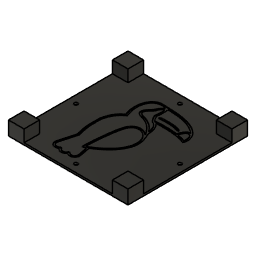
base (Autodesk Fusion 360 design; units mm, degrees)
Autodesk Fusion 360 part; units mm, degrees
sketch "Sketch1" plane through (0, 0, 0) normal (0, 0, 1) x (1, 0, 0)
  line L0 (-50, 50) -> (50, 50)
  line L1 (50, 50) -> (50, -50)
  line L2 (50, -50) -> (-50, -50)
  line L3 (-50, -50) -> (-50, 50)
  dimension "d73" = 100
  constraint horizontal L0
  constraint vertical L1
  constraint horizontal L2
  constraint vertical L3
  measures "d73" distance of L0.start L0.end
extrude "Extrude1" add sketch "Sketch1" along normal blind 1.6
sketch "Sketch2" plane through (0, 0, 1.6) normal (0, 0, 1) x (-1, 0, 0)
  line L0 (50, 50) -> (-50, 50)
  line L1 (-50, 50) -> (-50, -50)
  line L2 (-50, -50) -> (50, -50)
  line L3 (50, -50) -> (50, 50)
  line L4 (50, -50) -> (37, -50)
  line L5 (37, -50) -> (37, -37)
  line L6 (37, -37) -> (50, -37)
  line L7 (50, -37) -> (50, -50)
  dimension "d3" = 13
  dimension "d4" = 13
  constraint horizontal L4
  constraint vertical L5
  constraint horizontal L6
  constraint vertical L7
  constraint coincident L2.end L3.start
  measures "d3" distance of L2.end L4.end
  measures "d4" distance of L2.end L6.end
extrude "Extrude2" add sketch "Sketch2" along normal blind 10 contours L2 L3 L4 L5 L6 L7
sketch "Sketch3" plane through (0, 0, 1.6) normal (0, 0, 1) x (-1, 0, 0)
  line L0 (37, -50) -> (37, -37)
  line L1 (37, -37) -> (50, -37)
  line L2 (50, -37) -> (50, 50)
  line L3 (50, 50) -> (-50, 50)
  line L4 (-50, 50) -> (-50, -50)
  line L5 (-50, -50) -> (37, -50)
  line L6 (50, 50) -> (37, 50)
  line L7 (37, 50) -> (37, 37)
  line L8 (37, 37) -> (50, 37)
  line L9 (50, 37) -> (50, 50)
  dimension "d7" = 13
  dimension "d8" = 13
  constraint horizontal L6
  constraint vertical L7
  constraint horizontal L8
  constraint vertical L9
  constraint coincident L2.end L3.start
  measures "d7" distance of L2.end L6.end
  measures "d8" distance of L2.end L8.end
extrude "Extrude3" add sketch "Sketch3" along normal blind 10 contours L2 L3 L6 L7 L8 L9
sketch "Sketch4" plane through (0, 0, 1.6) normal (0, 0, 1) x (-1, 0, 0)
  line L0 (37, 37) -> (37, 50)
  line L1 (37, 50) -> (-50, 50)
  line L2 (-50, 50) -> (-50, -50)
  line L3 (-50, -50) -> (37, -50)
  line L4 (37, -50) -> (37, -37)
  line L5 (37, -37) -> (50, -37)
  line L6 (50, -37) -> (50, 37)
  line L7 (50, 37) -> (37, 37)
  line L8 (-50, 50) -> (-37, 50)
  line L9 (-37, 50) -> (-37, 37)
  line L10 (-37, 37) -> (-50, 37)
  line L11 (-50, 37) -> (-50, 50)
  dimension "d11" = 13
  dimension "d12" = 13
  constraint horizontal L8
  constraint vertical L9
  constraint horizontal L10
  constraint vertical L11
  constraint coincident L1.end L2.start
  measures "d11" distance of L1.end L8.end
  measures "d12" distance of L1.end L10.end
extrude "Extrude4" add sketch "Sketch4" along normal blind 10 contours L1 L2 L8 L9 L10 L11
sketch "Sketch5" plane through (0, 0, 1.6) normal (0, 0, 1) x (-1, 0, 0)
  line L0 (-37, 50) -> (-37, 37)
  line L1 (-37, 37) -> (-50, 37)
  line L2 (-50, 37) -> (-50, -50)
  line L3 (-50, -50) -> (37, -50)
  line L4 (37, -50) -> (37, -37)
  line L5 (37, -37) -> (50, -37)
  line L6 (50, -37) -> (50, 37)
  line L7 (50, 37) -> (37, 37)
  line L8 (37, 37) -> (37, 50)
  line L9 (37, 50) -> (-37, 50)
  line L10 (-50, -50) -> (-37, -50)
  line L11 (-37, -50) -> (-37, -37)
  line L12 (-37, -37) -> (-50, -37)
  line L13 (-50, -37) -> (-50, -50)
  dimension "d15" = 13
  dimension "d16" = 13
  constraint horizontal L10
  constraint vertical L11
  constraint horizontal L12
  constraint vertical L13
  constraint coincident L2.end L3.start
  measures "d15" distance of L2.end L10.end
  measures "d16" distance of L2.end L12.end
extrude "Extrude5" add sketch "Sketch5" along normal blind 10 contours L2 L3 L10 L11 L12 L13
sketch "Sketch15" plane through (0, 0, 1.6) normal (0, 0, 1) x (1, 0, 0)
  line L0 (-40, 50) -> (-50, 50)
  line L1 (-50, -50) -> (-40, -50)
  line L2 (-50, -40) -> (-50, -50)
  line L3 (50, -50) -> (50, -40)
  line L4 (40, -50) -> (50, -50)
  line L5 (50, 50) -> (40, 50)
  line L6 (-50, 50) -> (-50, 40)
  line L7 (50, 40) -> (50, 50)
  line L8 (40, 50) -> (-40, 50)
  line L9 (50, -40) -> (50, 40)
  line L10 (-40, -50) -> (40, -50)
  line L11 (-50, 40) -> (-50, -40)
  line L12 (37, 37) -> (37, 50)
  line L13 (37, 50) -> (-37, 50)
  line L14 (-37, 50) -> (-37, 37)
  line L15 (-37, 37) -> (-50, 37)
  line L16 (-50, 37) -> (-50, -37)
  line L17 (-50, -37) -> (-37, -37)
  line L18 (-37, -37) -> (-37, -50)
  line L19 (-37, -50) -> (37, -50)
  line L20 (37, -50) -> (37, -37)
  line L21 (37, -37) -> (50, -37)
  line L22 (50, -37) -> (50, 37)
  line L23 (50, 37) -> (37, 37)
  point P0 (-43.5004, 0.0001)
  point P1 (0.0001, 43.5004)
  point P2 (43.5004, -0.0001)
  point P3 (-0.0001, -43.5004)
  dimension "d36" = 50
  dimension "d38" = 50
  dimension "d40" = 50
  dimension "d43" = 50
  dimension "d45" = 6.5
  dimension "d47" = 6.5
  dimension "d49" = 6.5
  dimension "d51" = 6.5
  measures "d36" distance of P0 L0
  measures "d38" distance of P3 L2
  measures "d40" distance of P2 L4
  measures "d43" distance of P1 L7
  measures "d45" distance of P1 L8
  measures "d47" distance of P2 L9
  measures "d49" distance of P3 L10
  measures "d51" distance of P0 L11
hole "Hole1" at (-0.0001, -43.5004, 1.6711) at (-43.5004, 0.0001, 1.6711) at (43.5004, -0.0001, 1.6711) at (0.0001, 43.5004, 1.6711) direction (0, 0, -1) diameter 3 depth 15 tip angle 118
sketch "Sketch16" plane through (0, 0, 0) normal (0, 0, 1) x (1, 0, 0)
  spline S0 degree 3 poles (-9.4935, 35.6608) (-16.0287, 33.5706) (-18.8069, 24.1515) (-15.6848, 14.891) knots 0 0 0 0 1 1 1 1
  spline S1 degree 3 poles (-15.6848, 14.891) (-15.3673, 13.965) (-15.1292, 13.1977) (-15.1821, 13.1713) knots 0 0 0 0 1 1 1 1
  spline S2 degree 3 poles (-15.1821, 13.1713) (-18.5158, 10.9752) (-21.241, 6.8477) (-22.5904, 2.0323) knots 0 0 0 0 1 1 1 1
  spline S3 degree 3 poles (-22.5904, 2.0323) (-23.1196, 0.1537) (-23.1725, -0.7194) (-23.1725, -5.6406) knots 0 0 0 0 1 1 1 1
  spline S4 degree 3 poles (-23.1725, -5.6406) (-23.1725, -11.4615) (-22.9608, -13.3929) (-21.6115, -18.9227) knots 0 0 0 0 1 1 1 1
  line L0 (-21.6115, -18.9227) -> (-21.0029, -21.4627)
  line L1 (-21.0029, -21.4627) -> (-23.1196, -28.6065)
  spline S5 degree 3 poles (-23.1196, -28.6065) (-24.6277, -33.7129) (-25.1833, -35.9883) (-25.0775, -36.5704) knots 0 0 0 0 1 1 1 1
  spline S6 degree 3 poles (-25.0775, -36.5704) (-24.8394, -37.761) (-23.9927, -39.031) (-23.0137, -39.6396) knots 0 0 0 0 1 1 1 1
  spline S7 degree 3 poles (-23.0137, -39.6396) (-21.9554, -40.2746) (-19.7329, -40.354) (-18.9127, -39.7719) knots 0 0 0 0 1 1 1 1
  spline S8 degree 3 poles (-18.9127, -39.7719) (-18.3835, -39.4015) (-18.2777, -39.4279) (-17.5633, -40.1423) knots 0 0 0 0 1 1 1 1
  spline S9 degree 3 poles (-17.5633, -40.1423) (-15.9758, -41.7563) (-13.33, -41.7298) (-11.7954, -40.1423) knots 0 0 0 0 1 1 1 1
  spline S10 degree 3 poles (-11.7954, -40.1423) (-11.1075, -39.4279) (-11.0281, -39.4015) (-10.5783, -39.8248) knots 0 0 0 0 1 1 1 1
  spline S11 degree 3 poles (-10.5783, -39.8248) (-9.9433, -40.3804) (-7.6679, -40.5921) (-6.6625, -40.1688) knots 0 0 0 0 1 1 1 1
  spline S12 degree 3 poles (-6.6625, -40.1688) (-5.5512, -39.719) (-4.3342, -38.2373) (-4.1225, -37.0996) knots 0 0 0 0 1 1 1 1
  spline S13 degree 3 poles (-4.1225, -37.0996) (-3.9902, -36.4117) (-4.2283, -34.7448) (-4.9162, -31.4904) knots 0 0 0 0 1 1 1 1
  spline S14 degree 3 poles (-4.9162, -31.4904) (-5.4454, -28.9504) (-5.8423, -26.8338) (-5.8158, -26.8338) knots 0 0 0 0 1 1 1 1
  spline S15 degree 3 poles (-5.8158, -26.8338) (-5.7629, -26.8073) (-4.5458, -26.0135) (-3.0906, -25.0346) knots 0 0 0 0 1 1 1 1
  spline S16 degree 3 poles (-3.0906, -25.0346) (4.5029, -19.981) (9.7681, -13.4458) (11.3821, -7.0429) knots 0 0 0 0 1 1 1 1
  spline S17 degree 3 poles (11.3821, -7.0429) (12.1229, -4.0796) (11.9642, -0.296) (11.0117, 2.1646) knots 0 0 0 0 1 1 1 1
  spline S18 degree 3 poles (11.0117, 2.1646) (10.6148, 3.1171) (10.1915, 4.3606) (10.0063, 4.9427) knots 0 0 0 0 1 1 1 1
  spline S19 degree 3 poles (10.0063, 4.9427) (9.821, 5.5248) (9.3977, 6.5302) (9.0538, 7.1652) knots 0 0 0 0 1 1 1 1
  spline S20 degree 3 poles (9.0538, 7.1652) (8.6569, 7.906) (8.4188, 8.7527) (8.4188, 9.5465) knots 0 0 0 0 1 1 1 1
  spline S21 degree 3 poles (8.4188, 9.5465) (8.3923, 12.8008) (7.0165, 16.5315) (5.2173, 18.1719) knots 0 0 0 0 1 1 1 1
  spline S22 degree 3 poles (5.2173, 18.1719) (4.6088, 18.701) (4.1854, 19.2037) (4.2648, 19.2831) knots 0 0 0 0 1 1 1 1
  spline S23 degree 3 poles (4.2648, 19.2831) (4.3442, 19.336) (7.0165, 19.389) (10.1915, 19.389) knots 0 0 0 0 1 1 1 1
  spline S24 degree 3 poles (10.1915, 19.389) (17.8644, 19.389) (24.5054, 18.4894) (27.8656, 17.0077) knots 0 0 0 0 1 1 1 1
  spline S25 degree 3 poles (27.8656, 17.0077) (28.4742, 16.7431) (29.1092, 16.5844) (29.2679, 16.6902) knots 0 0 0 0 1 1 1 1
  spline S26 degree 3 poles (29.2679, 16.6902) (29.7442, 16.9812) (30.194, 19.6006) (30.0088, 21.0029) knots 0 0 0 0 1 1 1 1
  spline S27 degree 3 poles (30.0088, 21.0029) (29.1356, 27.4588) (22.4946, 32.4329) (12.0965, 34.3908) knots 0 0 0 0 1 1 1 1
  spline S28 degree 3 poles (12.0965, 34.3908) (8.604, 35.0788) (7.281, 35.211) (1.1427, 35.555) knots 0 0 0 0 1 1 1 1
  spline S29 degree 3 poles (1.1427, 35.555) (-7.5621, 36.0312) (-8.3294, 36.0312) (-9.4935, 35.6608) knots 0 0 0 0 1 1 1 1
  spline S30 degree 3 poles (-4.3342, 34.5496) (-2.9054, 34.3644) (-2.5879, 33.9675) (-3.3817, 33.3325) knots 0 0 0 0 1 1 1 1
  spline S31 degree 3 poles (-3.3817, 33.3325) (-4.8898, 32.1419) (-5.5777, 31.2423) (-6.1069, 29.7871) knots 0 0 0 0 1 1 1 1
  spline S32 degree 3 poles (-6.1069, 29.7871) (-6.5567, 28.57) (-7.0858, 27.8027) (-8.3029, 26.6121) knots 0 0 0 0 1 1 1 1
  spline S33 degree 3 poles (-8.3029, 26.6121) (-10.1815, 24.76) (-10.9487, 23.4106) (-10.9752, 21.8231) knots 0 0 0 0 1 1 1 1
  spline S34 degree 3 poles (-10.9752, 21.8231) (-11.0017, 19.7329) (-9.6787, 18.6217) (-6.1862, 17.7485) knots 0 0 0 0 1 1 1 1
  spline S35 degree 3 poles (-6.1862, 17.7485) (-2.535, 16.8225) (1.1163, 14.7588) (3.5504, 12.1658) knots 0 0 0 0 1 1 1 1
  spline S36 degree 3 poles (3.5504, 12.1658) (4.9263, 10.7371) (7.6779, 7.1652) (7.5192, 7.0065) knots 0 0 0 0 1 1 1 1
  spline S37 degree 3 poles (7.5192, 7.0065) (7.4663, 6.9535) (6.9106, 7.271) (6.2756, 7.6944) knots 0 0 0 0 1 1 1 1
  spline S38 degree 3 poles (6.2756, 7.6944) (4.7675, 8.7262) (2.1481, 9.4142) (0.5077, 9.176) knots 0 0 0 0 1 1 1 1
  spline S39 degree 3 poles (0.5077, 9.176) (-2.244, 8.7792) (-4.4665, 7.0858) (-5.71, 4.44) knots 0 0 0 0 1 1 1 1
  spline S40 degree 3 poles (-5.71, 4.44) (-7.6679, 0.286) (-9.2025, -10.2179) (-9.9962, -24.8758) knots 0 0 0 0 1 1 1 1
  spline S41 degree 3 poles (-9.9962, -24.8758) (-10.155, -27.9715) (-10.1285, -28.2625) (-9.7052, -28.4477) knots 0 0 0 0 1 1 1 1
  spline S42 degree 3 poles (-9.7052, -28.4477) (-9.3877, -28.5535) (-8.8321, -28.3948) (-8.1971, -28.0244) knots 0 0 0 0 1 1 1 1
  spline S43 degree 3 poles (-8.1971, -28.0244) (-7.4562, -27.601) (-7.1652, -27.5481) (-7.0858, -27.7863) knots 0 0 0 0 1 1 1 1
  spline S44 degree 3 poles (-7.0858, -27.7863) (-7.0329, -27.9715) (-6.6096, -30.0088) (-6.1598, -32.2842) knots 0 0 0 0 1 1 1 1
  spline S45 degree 3 poles (-6.1598, -32.2842) (-5.3925, -36.1206) (-5.3396, -36.5175) (-5.71, -37.3642) knots 0 0 0 0 1 1 1 1
  spline S46 degree 3 poles (-5.71, -37.3642) (-6.4773, -39.1633) (-8.6733, -39.6396) (-10.1815, -38.3167) knots 0 0 0 0 1 1 1 1
  spline S47 degree 3 poles (-10.1815, -38.3167) (-11.3192, -37.3377) (-11.5837, -37.3377) (-12.0865, -38.2902) knots 0 0 0 0 1 1 1 1
  spline S48 degree 3 poles (-12.0865, -38.2902) (-12.6156, -39.3485) (-13.4887, -39.9042) (-14.5471, -39.9042) knots 0 0 0 0 1 1 1 1
  spline S49 degree 3 poles (-14.5471, -39.9042) (-15.6583, -39.9042) (-16.9019, -39.2692) (-17.1135, -38.6077) knots 0 0 0 0 1 1 1 1
  spline S50 degree 3 poles (-17.1135, -38.6077) (-17.431, -37.5758) (-17.9073, -37.47) (-18.9656, -38.1844) knots 0 0 0 0 1 1 1 1
  spline S51 degree 3 poles (-18.9656, -38.1844) (-21.0294, -39.5867) (-23.5694, -38.5019) (-23.5958, -36.2) knots 0 0 0 0 1 1 1 1
  spline S52 degree 3 poles (-23.5958, -36.2) (-23.5958, -35.6973) (-22.6962, -32.1783) (-21.585, -28.3948) knots 0 0 0 0 1 1 1 1
  line L2 (-21.585, -28.3948) -> (-19.5742, -21.5156)
  line L3 (-19.5742, -21.5156) -> (-20.2356, -18.6052)
  spline S53 degree 3 poles (-20.2356, -18.6052) (-21.585, -12.9167) (-21.8496, -10.6942) (-21.8496, -5.5083) knots 0 0 0 0 1 1 1 1
  spline S54 degree 3 poles (-21.8496, -5.5083) (-21.8231, -1.3544) (-21.7437, -0.296) (-21.2675, 1.5031) knots 0 0 0 0 1 1 1 1
  spline S55 degree 3 poles (-21.2675, 1.5031) (-20.315, 4.9692) (-18.8069, 7.7208) (-16.6373, 9.9433) knots 0 0 0 0 1 1 1 1
  spline S56 degree 3 poles (-16.6373, 9.9433) (-15.579, 11.0017) (-14.4412, 12.0335) (-14.0708, 12.2717) knots 0 0 0 0 1 1 1 1
  line L4 (-14.0708, 12.2717) -> (-13.4094, 12.6685)
  line L5 (-13.4094, 12.6685) -> (-14.256, 15.1821)
  spline S57 degree 3 poles (-14.256, 15.1821) (-17.2723, 24.0721) (-14.8381, 32.724) (-8.8585, 34.3379) knots 0 0 0 0 1 1 1 1
  spline S58 degree 3 poles (-8.8585, 34.3379) (-7.4033, 34.7348) (-6.3185, 34.7612) (-4.3342, 34.5496) knots 0 0 0 0 1 1 1 1
  spline S59 degree 3 poles (10.4031, 33.2796) (15.5096, 32.38) (19.8488, 30.8454) (22.7592, 28.8875) knots 0 0 0 0 1 1 1 1
  spline S60 degree 3 poles (22.7592, 28.8875) (25.9342, 26.7708) (26.1458, 26.5062) (24.8229, 26.5062) knots 0 0 0 0 1 1 1 1
  spline S61 degree 3 poles (24.8229, 26.5062) (23.3148, 26.5062) (21.5685, 24.3896) (20.6954, 21.4792) knots 0 0 0 0 1 1 1 1
  line L6 (20.6954, 21.4792) -> (20.325, 20.2356)
  line L7 (20.325, 20.2356) -> (18.8169, 20.4473)
  spline S62 degree 3 poles (18.8169, 20.4473) (15.6683, 20.8971) (8.8156, 21.0294) (5.376, 20.7119) knots 0 0 0 0 1 1 1 1
  line L8 (5.376, 20.7119) -> (1.9629, 20.3944)
  line L9 (1.9629, 20.3944) -> (1.2221, 21.2675)
  spline S63 degree 3 poles (1.2221, 21.2675) (0.8252, 21.7437) (0.1902, 22.7492) (-0.1802, 23.4635) knots 0 0 0 0 1 1 1 1
  spline S64 degree 3 poles (-0.1802, 23.4635) (-0.7358, 24.6013) (-0.7887, 24.9452) (-0.5771, 25.8448) knots 0 0 0 0 1 1 1 1
  spline S65 degree 3 poles (-0.5771, 25.8448) (-0.2596, 27.1942) (-0.2331, 31.9302) (-0.5506, 33.0415) knots 0 0 0 0 1 1 1 1
  spline S66 degree 3 poles (-0.5506, 33.0415) (-0.6829, 33.4913) (-0.7623, 33.9146) (-0.7094, 33.9675) knots 0 0 0 0 1 1 1 1
  spline S67 degree 3 poles (-0.7094, 33.9675) (-0.4712, 34.1792) (8.3129, 33.65) (10.4031, 33.2796) knots 0 0 0 0 1 1 1 1
  spline S68 degree 3 poles (-1.6354, 30.0517) (-1.6354, 28.7817) (-1.7677, 27.0354) (-1.9265, 26.1358) knots 0 0 0 0 1 1 1 1
  spline S69 degree 3 poles (-1.9265, 26.1358) (-2.191, 24.7071) (-2.1646, 24.3896) (-1.6883, 23.3312) knots 0 0 0 0 1 1 1 1
  spline S70 degree 3 poles (-1.6883, 23.3312) (-0.9475, 21.6379) (1.1692, 18.9127) (1.8835, 18.7275) knots 0 0 0 0 1 1 1 1
  spline S71 degree 3 poles (1.8835, 18.7275) (2.9683, 18.4629) (4.6617, 17.0342) (5.4025, 15.7642) knots 0 0 0 0 1 1 1 1
  spline S72 degree 3 poles (5.4025, 15.7642) (6.0375, 14.6794) (7.2281, 10.6842) (6.99, 10.446) knots 0 0 0 0 1 1 1 1
  spline S73 degree 3 poles (6.99, 10.446) (6.9371, 10.3931) (6.5931, 10.7635) (6.1963, 11.2927) knots 0 0 0 0 1 1 1 1
  spline S74 degree 3 poles (6.1963, 11.2927) (3.0477, 15.3937) (-1.4502, 18.1454) (-7.2446, 19.4683) knots 0 0 0 0 1 1 1 1
  spline S75 degree 3 poles (-7.2446, 19.4683) (-8.4617, 19.7329) (-9.5729, 20.8971) (-9.5729, 21.8496) knots 0 0 0 0 1 1 1 1
  spline S76 degree 3 poles (-9.5729, 21.8496) (-9.5729, 22.9608) (-8.3558, 24.8394) (-6.8477, 26.0829) knots 0 0 0 0 1 1 1 1
  spline S77 degree 3 poles (-6.8477, 26.0829) (-5.9217, 26.8237) (-5.4983, 27.4588) (-5.075, 28.57) knots 0 0 0 0 1 1 1 1
  spline S78 degree 3 poles (-5.075, 28.57) (-4.2812, 30.7925) (-4.0167, 31.2158) (-3.1171, 31.7979) knots 0 0 0 0 1 1 1 1
  spline S79 degree 3 poles (-3.1171, 31.7979) (-1.7412, 32.671) (-1.6354, 32.5652) (-1.6354, 30.0517) knots 0 0 0 0 1 1 1 1
  spline S80 degree 3 poles (26.7808, 24.8658) (27.7333, 24.4425) (28.5271, 22.22) (28.5271, 19.9975) knots 0 0 0 0 1 1 1 1
  spline S81 degree 3 poles (28.5271, 19.9975) (28.5271, 18.4365) (28.4742, 18.2777) (28.0773, 18.4629) knots 0 0 0 0 1 1 1 1
  spline S82 degree 3 poles (28.0773, 18.4629) (27.1777, 18.8333) (23.1031, 19.8652) (22.3623, 19.8652) knots 0 0 0 0 1 1 1 1
  spline S83 degree 3 poles (22.3623, 19.8652) (21.4892, 19.8917) (21.5156, 20.0504) (22.6533, 22.6169) knots 0 0 0 0 1 1 1 1
  spline S84 degree 3 poles (22.6533, 22.6169) (23.6852, 24.9717) (25.0081, 25.686) (26.7808, 24.8658) knots 0 0 0 0 1 1 1 1
  spline S85 degree 3 poles (4.2383, 7.1917) (6.2227, 6.4508) (8.2335, 4.5987) (9.2125, 2.6144) knots 0 0 0 0 1 1 1 1
  spline S86 degree 3 poles (9.2125, 2.6144) (11.6996, -2.4656) (10.5619, -8.6569) (5.9846, -14.8217) knots 0 0 0 0 1 1 1 1
  spline S87 degree 3 poles (5.9846, -14.8217) (4.1854, -17.2558) (-0.3125, -21.4892) (-3.1171, -23.3942) knots 0 0 0 0 1 1 1 1
  spline S88 degree 3 poles (-3.1171, -23.3942) (-5.6571, -25.114) (-8.4881, -26.7808) (-8.6204, -26.6485) knots 0 0 0 0 1 1 1 1
  spline S89 degree 3 poles (-8.6204, -26.6485) (-8.7792, -26.4633) (-8.0119, -15.536) (-7.5885, -11.726) knots 0 0 0 0 1 1 1 1
  spline S90 degree 3 poles (-7.5885, -11.726) (-6.8477, -5.0321) (-5.6306, 1.0798) (-4.5987, 3.514) knots 0 0 0 0 1 1 1 1
  spline S91 degree 3 poles (-4.5987, 3.514) (-3.8844, 5.1279) (-2.535, 6.636) (-1.2385, 7.2181) knots 0 0 0 0 1 1 1 1
  spline S92 degree 3 poles (-1.2385, 7.2181) (0.1638, 7.8796) (2.4656, 7.8531) (4.2383, 7.1917) knots 0 0 0 0 1 1 1 1
  spline S93 degree 3 poles (3.3652, 25.4744) (1.6983, 25.2362) (1.275, 25.051) (1.275, 24.5219) knots 0 0 0 0 1 1 1 1
  spline S94 degree 3 poles (1.275, 24.5219) (1.275, 23.8869) (1.7248, 23.834) (5.085, 24.1515) knots 0 0 0 0 1 1 1 1
  spline S95 degree 3 poles (5.085, 24.1515) (8.6833, 24.4954) (13.1813, 24.2044) (15.8271, 23.4635) knots 0 0 0 0 1 1 1 1
  spline S96 degree 3 poles (15.8271, 23.4635) (16.6208, 23.2254) (17.7321, 22.9873) (18.2877, 22.8815) knots 0 0 0 0 1 1 1 1
  spline S97 degree 3 poles (18.2877, 22.8815) (19.2402, 22.7492) (19.3196, 22.7756) (19.2138, 23.3312) knots 0 0 0 0 1 1 1 1
  spline S98 degree 3 poles (19.2138, 23.3312) (19.1344, 24.0192) (18.2348, 24.3896) (15.2979, 25.0775) knots 0 0 0 0 1 1 1 1
  spline S99 degree 3 poles (15.2979, 25.0775) (13.3135, 25.5273) (5.6142, 25.7919) (3.3652, 25.4744) knots 0 0 0 0 1 1 1 1
  spline S100 degree 3 poles (-20.2356, -45.6456) (-9.2819, -45.6985) (8.6569, -45.6985) (19.5842, -45.6456) knots 0 0 0 0 1 1 1 1
  spline S101 degree 3 poles (19.5842, -45.6456) (30.5379, -45.6192) (21.595, -45.5927) (-0.3125, -45.5927) knots 0 0 0 0 1 1 1 1
  spline S102 degree 3 poles (-0.3125, -45.5927) (-22.22, -45.5927) (-31.1629, -45.6192) (-20.2356, -45.6456) knots 0 0 0 0 1 1 1 1
emboss "Emboss1" depth -0.5 profiles "Sketch16" section 1 contours S0 S1 S2 S3 S4 L0 L1 S5 S6 S7 S8 S9 S10 S11 S12 S13 S14 S15 S16 S17 S18 S19 S20 S21 S22 S23 S24 S25 S26 S27 S28 S29 | S93 S94 S95 S96 S97 S98 S99 onto face at (-14.0023, -0.0461, 1.6)
sketch "Sketch17" plane through (0, 0, 0) normal (0, 0, -1) x (1, 0, 0)
  circle A0 centre (43.5004, 0.0001) radius 1.5
  circle A1 centre (-0.0001, 43.5004) radius 1.5
  circle A2 centre (-43.5004, -0.0001) radius 1.5
  circle A3 centre (0.0001, -43.5004) radius 1.5
  line L0 (50, 50) -> (-50, 50)
  line L1 (-50, 50) -> (-50, -50)
  line L2 (-50, -50) -> (50, -50)
  line L3 (50, -50) -> (50, 50)
  circle A4 centre (-42.5, 42.5) radius 4
  circle A5 centre (42.5, 42.5) radius 4
  circle A6 centre (-42.5, -42.5) radius 4
  circle A7 centre (42.5, -42.5) radius 4
  point P0 (-42.5, 42.5)
  point P1 (42.5, 42.5)
  point P2 (-42.5, -42.5)
  point P3 (42.5, -42.5)
  dimension "d59" = 7.5
  dimension "d60" = 7.5
  dimension "d61" = 7.5
  dimension "d62" = 7.5
  dimension "d63" = 7.5
  dimension "d64" = 7.5
  dimension "d65" = 7.5
  dimension "d66" = 7.5
  dimension "d67" = 8
  dimension "d68" = 8
  dimension "d69" = 8
  dimension "d70" = 8
  constraint coincident P0 A4.centre
  constraint coincident P1 A5.centre
  constraint coincident P2 A6.centre
  constraint coincident P3 A7.centre
  measures "d59" distance of L2 P2
  measures "d60" distance of L2 P3
  measures "d61" distance of L0 P0
  measures "d62" distance of L0 P1
  measures "d63" distance of L3 P1
  measures "d64" distance of L1 P0
  measures "d65" distance of L3 P3
  measures "d66" distance of L1 P2
  measures "d67" diameter of A4
  measures "d68" diameter of A5
  measures "d69" diameter of A6
  measures "d70" diameter of A7
sketch "Sketch18" plane through (0, 0, 0) normal (0, 0, -1) x (1, 0, 0)
extrude "Extrude9" cut sketch "Sketch17" against normal blind 6.5 contours A4 | A5 | A6 | A7
